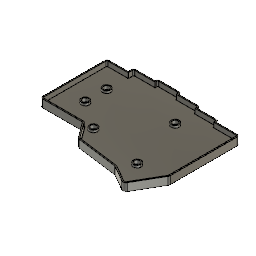
dubu36-travel-case (Autodesk Fusion 360 archive; units mm, degrees)
design "Corne Slim Case"
Autodesk Fusion 360 part; units mm, degrees
sketch "Corne PCB" plane through (-57.8876, 153.4022, 0) normal (0, 0, 1) x (1, 0, 0)
  arc A0 (136, -62.75) -> (136.5, -63.25) centre (136.5, -62.75) ccw
  arc A1 (117.5, -63.25) -> (118, -62.75) centre (117.5, -62.75) ccw
  arc A2 (80, -123.75) -> (80.5, -124.25) centre (80.5, -123.75) ccw
  arc A3 (99.5, -63.25) -> (99, -63.75) centre (99.5, -63.75) ccw
  arc A4 (98.5, -68) -> (99, -67.5) centre (98.5, -67.5) ccw
  arc A5 (80.5, -68) -> (80, -68.5) centre (80.5, -68.5) ccw
  arc A6 (136, -61.5) -> (135.5, -61) centre (135.5, -61.5) ccw
  arc A7 (118.5, -61) -> (118, -61.5) centre (118.5, -61.5) ccw
  arc A8 (165.0746, -143.8996) -> (164.4202, -143.7699) centre (164.087, -147.168) ccw
  line L0 (116.8536, -124.3964) -> (127.3964, -138.8536)
  arc A9 (179.369, -152.161) -> (181.297, -151.7815) centre (180.144, -151.011) ccw
  arc A10 (174, -66.25) -> (173.5, -65.75) centre (173.5, -66.25) ccw
  line L1 (174, -66.25) -> (174, -67.5)
  arc A11 (127.3964, -138.8536) -> (127.75, -139) centre (127.75, -138.5) ccw
  arc A12 (194.523, -128.848) -> (194.75, -127.9616) centre (193.048, -127.998) ccw
  line L2 (127.75, -139) -> (164.4202, -143.7699)
  arc A13 (116.8536, -124.3964) -> (116.5, -124.25) centre (116.5, -124.75) ccw
  line L3 (194.75, -68.5) -> (194.75, -127.9616)
  arc A14 (155, -65.25) -> (155.5, -65.75) centre (155.5, -65.25) ccw
  arc A15 (155, -63.75) -> (154.5, -63.25) centre (154.5, -63.75) ccw
  arc A16 (194.75, -68.5) -> (194.25, -68) centre (194.25, -68.5) ccw
  line L4 (116.5, -124.25) -> (80.5, -124.25)
  line L5 (181.297, -151.7815) -> (194.523, -128.848)
  line L6 (194.25, -68) -> (174.5, -68)
  arc A17 (174, -67.5) -> (174.5, -68) centre (174.5, -67.5) ccw
  line L7 (165.0746, -143.8996) -> (179.369, -152.161)
  line L8 (118, -61.5) -> (118, -62.75)
  line L9 (135.5, -61) -> (118.5, -61)
  circle A18 centre (122.75, -122.75) radius 2.45
  line L10 (117.5, -63.25) -> (99.5, -63.25)
  circle A19 centre (98.5, -86.75) radius 2.45
  line L11 (136, -62.75) -> (136, -61.5)
  circle A20 centre (155.5, -83) radius 2.45
  circle A21 centre (169.25, -130.5) radius 2.45
  line L12 (155, -65.25) -> (155, -63.75)
  line L13 (98.5, -68) -> (80.5, -68)
  circle A22 centre (98.5, -105.75) radius 2.45
  line L14 (154.5, -63.25) -> (136.5, -63.25)
  line L15 (99, -63.75) -> (99, -67.5)
  line L16 (173.5, -65.75) -> (155.5, -65.75)
  arc A23 (80, -89.1484) -> (80, -84.3516) centre (79.5, -86.75) ccw
  arc A24 (80, -107.8984) -> (80, -103.1016) centre (79.5, -105.5) ccw
  line L17 (80, -107.8984) -> (80, -123.75)
  line L18 (80, -103.1016) -> (80, -89.1484)
  line L19 (80, -84.3516) -> (80, -68.5)
  line L20 (80, -84.3516) -> (80, -89.1484)
  line L21 (80, -103.1016) -> (80, -107.8984)
  dimension "d13" = 4.9
  dimension "d14" = 4.9
  dimension "d15" = 4.9
  dimension "d16" = 4.9
  dimension "d17" = 4.9
  constraint tangent A2 L17
  constraint parallel L17 L18
  constraint tangent A5 L19
  constraint coincident A12.start L5.end
  constraint coincident A12.end L3.end
  constraint coincident A9.end L5.start
  constraint coincident A9.start L7.end
  constraint coincident A8.start L7.start
  constraint coincident A8.end L2.end
  constraint coincident L0.end A11.start
  constraint coincident L0.start A13.start
  constraint horizontal L4
  constraint horizontal L13
  constraint horizontal L10
  constraint horizontal L9
  constraint horizontal L14
  constraint horizontal L16
  constraint horizontal L6
  constraint vertical L3
  constraint parallel L18 L20
  constraint parallel L17 L21
  measures "d13" diameter of A19
  measures "d14" diameter of A22
  measures "d15" diameter of A18
  measures "d16" diameter of A20
  measures "d17" diameter of A21
extrude "Extrude1" add sketch "Corne PCB" along normal blind 2 contours A0 A1 A2 A3 A4 A5 A6 A7 A8 L0 A9 A10 L1 A11 A12 L2 A13 L3 A14 A15 A16 L4 L5 L6 A17 L7 L8 L9 L10 L11 L12 L13 L14 L15 L16 A23 A24 L17 L18 L19 | A23 L20 | A24 L21 | A18 | A19 | A20 | A21 | A22
extrude "Extrude5" add sketch "Corne PCB" along normal blind 3
extrude "Extrude3" add sketch "Corne PCB" along normal blind 5 thin wall 1 outside contours A18 | A19 | A20 | A21 | A22
extrude "Extrude2" add sketch "Corne PCB" along normal blind 7 thin wall 1.5 outside contours A0 A1 A2 A3 A4 A5 A6 A7 A8 L0 A9 A10 L1 A11 A12 L2 A13 L3 A14 A15 A16 L4 L5 L6 A17 L7 L8 L9 L10 L11 L12 L13 L14 L15 L16 A23 A24 L17 L18 L19 | A23 L20 | A24 L21 | A18 | A19 | A20 | A21 | A22
extrude "Extrude6" cut sketch "Corne PCB" along normal blind 6 from surface at 2 thin wall 0.4 outside contours A0 A1 A2 A3 A4 A5 A6 A7 A8 L0 A9 A10 L1 A11 A12 L2 A13 L3 A14 A15 A16 L4 L5 L6 A17 L7 L8 L9 L10 L11 L12 L13 L14 L15 L16 A23 A24 L17 L18 L19 | A23 L20 | A24 L21 | A18 | A19 | A20 | A21 | A22
sketch "Switch Mounts" plane through (-57.8467, 153.3873, 0) normal (0, 0, 1) x (1, 0, 0)
  line L0 (170.188, -139.047) -> (182.312, -146.047)
  line L1 (189.312, -133.923) -> (177.188, -126.923)
  line L2 (177.188, -126.923) -> (170.188, -139.047)
  line L3 (152.542, -124.171) -> (148.919, -137.694)
  line L4 (162.442, -141.317) -> (166.065, -127.794)
  line L5 (129.53, -123.035) -> (129.53, -137.035)
  line L6 (148.919, -137.694) -> (162.442, -141.317)
  line L7 (166.065, -127.794) -> (152.542, -124.171)
  line L8 (129.53, -137.035) -> (143.53, -137.035)
  line L9 (182.312, -146.047) -> (189.312, -133.923)
  line L10 (82.01, -84.125) -> (96.01, -84.125)
  line L11 (82.01, -70.125) -> (82.01, -84.125)
  line L12 (134.01, -82) -> (120.01, -82)
  line L13 (172.01, -81.75) -> (172.01, -67.75)
  line L14 (172.01, -67.75) -> (158.01, -67.75)
  line L15 (120.01, -115) -> (134.01, -115)
  line L16 (82.01, -103.125) -> (96.01, -103.125)
  line L17 (172.01, -86.75) -> (158.01, -86.75)
  line L18 (101.01, -103.375) -> (101.01, -117.375)
  line L19 (139.01, -117.375) -> (153.01, -117.375)
  line L20 (115.01, -84.375) -> (101.01, -84.375)
  line L21 (115.01, -103.375) -> (101.01, -103.375)
  line L22 (153.01, -84.375) -> (139.01, -84.375)
  line L23 (158.01, -100.75) -> (172.01, -100.75)
  line L24 (101.01, -98.375) -> (115.01, -98.375)
  line L25 (134.01, -63) -> (120.01, -63)
  line L26 (158.01, -67.75) -> (158.01, -81.75)
  line L27 (139.01, -103.375) -> (139.01, -117.375)
  line L28 (139.01, -79.375) -> (153.01, -79.375)
  line L29 (120.01, -96) -> (134.01, -96)
  line L30 (115.01, -117.375) -> (115.01, -103.375)
  line L31 (158.01, -86.75) -> (158.01, -100.75)
  line L32 (153.01, -117.375) -> (153.01, -103.375)
  line L33 (139.01, -84.375) -> (139.01, -98.375)
  line L34 (115.01, -65.375) -> (101.01, -65.375)
  line L35 (96.01, -84.125) -> (96.01, -70.125)
  line L36 (120.01, -82) -> (120.01, -96)
  line L37 (96.01, -70.125) -> (82.01, -70.125)
  line L38 (134.01, -96) -> (134.01, -82)
  line L39 (139.01, -98.375) -> (153.01, -98.375)
  line L40 (101.01, -117.375) -> (115.01, -117.375)
  line L41 (96.01, -103.125) -> (96.01, -89.125)
  line L42 (134.01, -115) -> (134.01, -101)
  line L43 (82.01, -122.125) -> (96.01, -122.125)
  line L44 (172.01, -105.75) -> (158.01, -105.75)
  line L45 (82.01, -89.125) -> (82.01, -103.125)
  line L46 (158.01, -81.75) -> (172.01, -81.75)
  line L47 (153.01, -65.375) -> (139.01, -65.375)
  line L48 (101.01, -65.375) -> (101.01, -79.375)
  line L49 (158.01, -119.75) -> (172.01, -119.75)
  line L50 (153.01, -103.375) -> (139.01, -103.375)
  line L51 (143.53, -123.035) -> (129.53, -123.035)
  line L52 (120.01, -101) -> (120.01, -115)
  line L53 (153.01, -98.375) -> (153.01, -84.375)
  line L54 (120.01, -63) -> (120.01, -77)
  line L55 (101.01, -84.375) -> (101.01, -98.375)
  line L56 (172.01, -119.75) -> (172.01, -105.75)
  line L57 (82.01, -108.125) -> (82.01, -122.125)
  line L58 (120.01, -77) -> (134.01, -77)
  line L59 (96.01, -122.125) -> (96.01, -108.125)
  line L60 (153.01, -79.375) -> (153.01, -65.375)
  line L61 (96.01, -89.125) -> (82.01, -89.125)
  line L62 (172.01, -100.75) -> (172.01, -86.75)
  line L63 (96.01, -108.125) -> (82.01, -108.125)
  line L64 (134.01, -77) -> (134.01, -63)
  line L65 (134.01, -101) -> (120.01, -101)
  line L66 (158.01, -105.75) -> (158.01, -119.75)
  line L67 (101.01, -79.375) -> (115.01, -79.375)
  line L68 (115.01, -98.375) -> (115.01, -84.375)
  line L69 (143.53, -137.035) -> (143.53, -123.035)
  line L70 (139.01, -65.375) -> (139.01, -79.375)
  line L71 (115.01, -79.375) -> (115.01, -65.375)
  dimension "d28" = 14
  dimension "d29" = 14
  measures "d28" distance of L10.start L11.start
  measures "d29" distance of L11.start L35.end
